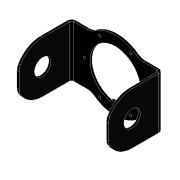
# Autodesk Inventor part: edge_j4-5
Saved by Autodesk Inventor 2022 (Build 260153000, 153)
## iProperties
Created: 2021-07-25
Part Number: edge_j4-5
Material: アルミニウム 6061
Document SubType Name: Sheet Metal
Designer: yuto6
Density: 2.7 g/cm^3
Sheet Metal Rule: Default_mm
Appearance: 滑らか - 黒
購入先: Meviy
在庫数: 0.0
Author: yuto6
Autodesk Inventor part; units mm, degrees
ref_plane "YZ Plane" through (0, 0, 0) normal (1, 0, 0) x (0, 1, 0)
ref_plane "XZ Plane" through (0, 0, 0) normal (0, 1, 0) x (-1, 0, 0)
ref_plane "XY Plane" through (0, 0, 0) normal (0, 0, 1) x (1, 0, 0)
sketch "スケッチ1" plane through (0, 0, 0) normal (0, 0, 1) x (1, 0, 0)
  line L0 (44.4, 25) -> (-44.4, 25)
  line L1 (-44.4, 25) -> (-44.4, -25)
  line L2 (-44.4, -25) -> (44.4, -25)
  line L3 (44.4, -25) -> (44.4, 25)
  line L4 (44.4, 25) -> (-44.4, -25) construction
  line L5 (-44.4, 25) -> (44.4, -25) construction
  point P0 (0, 0)
  dimension "d0" = 50
  dimension "d1" = 88.8
  measures "d0" distance of L0.end L1.end
  measures "d1" distance of L0.start L0.end
extrude "プレート1" add sketch "スケッチ1" along normal mid plane 2
sketch "スケッチ6" plane through (0, 0, -1) normal (0, 0, -1) x (-1, 0, 0)
  circle A0 centre (0, 0) radius 34
  dimension "d48" = 68
  constraints: 1 centre point, 1 coincident
  measures "d48" diameter of A0
extrude "押し出し2" add sketch "スケッチ6" against normal up to surface (2 mm away)
sketch "スケッチ2" plane through (42.4, 25, -1) normal (1, 0, 0) x (0, 1, 0)
  line L0 (-50, 0) -> (0, 0)
  line L1 (0, 0) -> (0, 55)
  line L2 (0, 55) -> (-50, 55)
  line L3 (-50, 55) -> (-50, 0)
  constraints: 6 end point, 1 horizontal, 1 perpendicular, 1 vertical
edge flange "フランジ1" height 55 angle 90 thickness 2 bend radius 2 thickness toward (1, 0, 0) relief tear relief width 2 relief depth 1 corner gap 2 corner form 0 edges at (44.4, 0, 1) (-44.4, 0, 1) wall of the first edge with corners at (42.4, -25, -1) (42.4, 25, -1) (42.4, 25, 54) (42.4, -25, 54)
bend "曲げ1"
corner "コーナー1"
fillet "フィレット1" radius 25 4 edges at (43.4, -25, 54) (-43.4, -25, 54) (-43.4, 25, 54) (43.4, 25, 54)
sketch "スケッチ3" plane through (44.4, -25, 3) normal (1, 0, 0) x (0, 0, -1)
  arc A0 (-26, 50) -> (-26, 0) centre (-26, 25) ccw projected
  point P0 (3, 25)
  point P1 (-26, 25)
  point P2 (-38, 25)
  point P3 (-26, 13)
  point P4 (-14, 25)
  point P5 (-26, 37)
  dimension "d24" = 360
  dimension "d52" = 12
  constraints: 1 coincident, 5 other
  measures "d52" distance of point (-26, 13) A0.centre
hole "穴1" at (44.4, 0, 29) direction (-1, 0, 0) diameter 16 end through all
sketch "スケッチ4" plane through (0, 0, -1) normal (0, 0, -1) x (-1, 0, 0)
  circle A0 centre (0, 0) radius 24.5
  dimension "d33" = 49
  constraints: 1 centre point, 1 coincident
  measures "d33" diameter of A0
extrude "押し出し1" cut sketch "スケッチ4" against normal through all
sketch "スケッチ5" plane through (0, 0, -1) normal (0, 0, -1) x (-1, 0, 0)
  point P0 (0, 0)
  point P1 (-30, 0)
  point P2 (-15, -25.9808)
  point P3 (15, -25.9808)
  point P4 (30, 0)
  point P5 (15, 25.9808)
  point P6 (-15, 25.9808)
  dimension "d36" = 30
  dimension "d39" = 360
  constraints: 7 other
  measures "d36" distance of point (0, 0) point (-30, 0)
hole "穴3" at (30, 0, -1) at (15, -25.9808, -1) at (-15, -25.9808, -1) at (-30, 0, -1) at (-15, 25.9808, -1) at (15, 25.9808, -1) direction (0, 0, 1) diameter 2.459 end through all thread size "M3x0.5" class "6H" standard "ANSI Metric M Profile"
fillet "コーナーR1" radius 12 4 edges at (23.0434, 25, 0) (-23.0434, 25, 0) (-23.0434, -25, 0) (23.0434, -25, 0)
sketch "スケッチ7" plane through (44.4, -25, 3) normal (1, 0, 0) x (0, 0, -1)
  line L0 (-49, 0) -> (-51, 0)
  line L1 (-51, 0) -> (-51, 50)
  line L2 (-51, 50) -> (-49, 50)
  line L3 (-49, 50) -> (-49, 0)
  arc A0 (-26, 50) -> (-26, 0) centre (-26, 25) ccw projected
  arc A1 (-26, 50) -> (-26, 0) centre (-26, 25) ccw projected
  point P0 (3, 25)
  dimension "d53" = 23
  constraints: 8 end point, 3 tangent, 2 parallel, 1 horizontal, 1 perpendicular
  measures "d53" distance from line of L3 A0.centre
extrude "押し出し3" cut sketch "スケッチ7" against normal through all
fillet "コーナーR2" radius 10 4 edges at (-43.4, 9.798, 52) (-43.4, -9.798, 52) (43.4, 9.798, 52) (43.4, -9.798, 52)
sketch "スケッチ8" plane through (0, 0, 1) normal (0, 0, 1) x (1, 0, 0)
  circle A0 centre (0, 0) radius 24.5 projected
  circle A1 centre (0, 0) radius 22.5
  line L0 (0, 0) -> (-4.2544, -24.1278)
  line L1 (0, 0) -> (4.2544, -24.1278)
  line L2 (0, 47.6) -> (0, -47.6) projected
  point P0 (-3.9071, -22.1582)
  point P1 (3.9071, -22.1582)
  dimension "d57" = 2
  dimension "d58" = 10
  dimension "d59" = 10
  constraints: 4 end point, 2 point on circle, 1 centre point
  measures "d57" radial gap between concentric circles of A0 A1
  measures "d58" angle of L2 L1
  measures "d59" angle of L0 L2
extrude "押し出し4" add sketch "スケッチ8" against normal up to surface (2 mm away) contours A0 L2 A1 L1 | A0 L0 A1 L2 picked at (3.2369, -23.6033) picked at (-3.6686, -23.5401)
fillet "コーナーR3" radius 0.5 4 edges at (-4.2544, -24.1278, 0) (-3.9071, -22.1582, 0) (3.9071, -22.1582, 0) (4.2544, -24.1278, 0)
equation "\"d13\" = 0.5 * d0"
equation "\"d46\" = Thickness"
equation "\"d2\" = Thickness"
equation "\"d3\" = BendReliefWidth"
equation "\"d4\" = BendReliefDepth"
equation "\"d5\" = MinimumRemnant"
equation "\"d6\" = TransitionRadius"
equation "\"d9\" = BendRadius"
equation "\"d10\" = CornerReliefSize"
equation "\"d11\" = GapSize"
equation "\"d12\" = JacobiRadiusSize"
equation "\"BendRadius\" = Thickness"
equation "\"BendReliefWidth\" = Thickness"
equation "\"BendReliefDepth\" = 0.5 * Thickness"
equation "\"CornerReliefSize\" = 4 * Thickness"
equation "\"MinimumRemnant\" = 2 * Thickness"
equation "\"TransitionRadius\" = BendRadius"
equation "\"JacobiRadiusSize\" = BendRadius"
equation "\"GapSize\" = Thickness"
equation "\"Thickness\" = 2"
